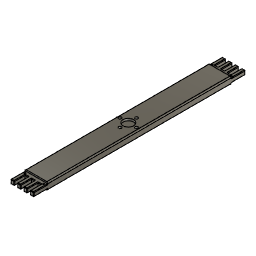
torsionbar_vFINAL v5 (Autodesk Fusion 360 design; units mm, degrees)
Autodesk Fusion 360 part; units mm, degrees
(part 1 of 5)
sketch "Sketch1" plane through (0, 0, 0) normal (0, 0, 1) x (1, 0, 0)
  line L0 (-15.999, -0.4) -> (-15.9943, 152)
  line L1 (16.0057, -0.4) -> (16.0057, 152)
  line L2 (16.0057, -0.4) -> (-15.999, -0.4)
  line L3 (-15.999, -0.4) -> (-15.9943, -152.8)
  line L4 (-15.9943, -152.8) -> (16.0057, -152.8)
  line L5 (16.0057, -0.4) -> (16.0057, -152.8)
  line L6 (16.0057, 152) -> (0.0057, 152)
  line L7 (0.0057, 152) -> (-15.9943, 152)
  dimension "d20" = 152.4
  dimension "d22" = 152.4
  dimension "d67" = 16
  dimension "d68" = 16
  constraint horizontal L2
  constraint symmetric L0.start L2 L3.start
  constraint symmetric L0.end L2 L3.end
  constraint symmetric L1.start L2 L5.start
  constraint symmetric L1.end L2 L4.end
  constraint vertical L1
  constraint perpendicular L1 L6
  constraint parallel L6 L7
  measures "d20" vertical distance of L0.start L0.end
  measures "d22" vertical distance of L1.start L1.end
  measures "d67" distance of L1.end L6.end
  measures "d68" distance of L0.end L6.end
extrude "Extrude3" add sketch "Sketch1" along normal blind 10
sketch "Sketch4" plane through (0, 0, 10) normal (0, 0, 1) x (-1, 0, 0)
  line L0 (15.999, 0.4) -> (15.9943, 152.8)
  line L1 (15.9943, 152.8) -> (-16.0057, 152.8)
  line L2 (-16.0057, 152.8) -> (-16.0057, -152)
  line L3 (15.9943, -152) -> (15.999, 0.4)
  circle A0 centre (0, 0) radius 7.5
  circle A1 centre (0, 11.5) radius 2
  circle A2 centre (-11.5, 0) radius 2
  circle A3 centre (0, -11.5) radius 2
  circle A4 centre (11.5, 0) radius 2
  line L4 (-16.0057, -152) -> (15.9943, -152)
  dimension "d36" = 15
  dimension "d50" = 4
  dimension "d51" = 4
  dimension "d52" = 4
  dimension "d53" = 4
  dimension "d54" = 11.5
  dimension "d55" = 11.5
  dimension "d56" = 11.5
  dimension "d57" = 11.5
  constraint coincident A0.centre origin
  measures "d36" diameter of A0
  measures "d50" diameter of A1
  measures "d51" diameter of A2
  measures "d52" diameter of A3
  measures "d53" diameter of A4
  measures "d54" distance of A0.centre A1.centre
  measures "d55" distance of A0.centre A4.centre
  measures "d56" distance of A0.centre A3.centre
  measures "d57" distance of A0.centre A2.centre
extrude "Extrude7" cut sketch "Sketch4" against normal blind 3 contours A0
extrude "Extrude9" cut sketch "Sketch4" against normal up to surface (10 mm away) contours A1 | A2 | A3 | A4
sketch "Sketch6" plane through (0, 152, 0) normal (0, 1, 0) x (-1, 0, 0)
  line L0 (-16.0057, 0) -> (15.9943, 0)
  line L1 (15.9943, 0) -> (15.9943, 10)
  line L2 (15.9943, 10) -> (-16.0057, 10)
  line L3 (-16.0057, 10) -> (-16.0057, 0)
  line L4 (10.9943, 8) -> (6.9943, 8)
  line L5 (1.9943, 8) -> (-2.0057, 8)
  line L6 (-7.0057, 8) -> (-11.0057, 8)
  line L7 (10.9943, 8) -> (10.9943, 2)
  line L8 (10.9943, 2) -> (6.9943, 2)
  line L9 (6.9943, 2) -> (6.9943, 8)
  line L10 (1.9943, 8) -> (1.9943, 2)
  line L11 (1.9943, 2) -> (-2.0057, 2)
  line L12 (-2.0057, 2) -> (-2.0057, 8)
  line L13 (-7.0057, 8) -> (-7.0057, 2)
  line L14 (-7.0057, 2) -> (-11.0057, 2)
  line L15 (-11.0057, 2) -> (-11.0057, 8)
  dimension "d78" = 4
  dimension "d79" = 4
  dimension "d80" = 4
  dimension "d95" = 6
  dimension "d96" = 4
  dimension "d97" = 4
  dimension "d98" = 4
  dimension "d99" = 5
  dimension "d100" = 5
  dimension "d101" = 2
  dimension "d102" = 2
  constraint perpendicular L4 L7
  constraint perpendicular L7 L8
  constraint perpendicular L5 L10
  constraint perpendicular L10 L11
  constraint perpendicular L6 L13
  constraint perpendicular L13 L14
  measures "d78" distance of L6.start L6.end
  measures "d79" distance of L5.start L5.end
  measures "d80" distance of L4.start L4.end
  measures "d95" distance of L4.start L7.end
  measures "d96" distance of L7.end L8.end
  measures "d97" distance of L10.end L11.end
  measures "d98" distance of L13.end L14.end
  measures "d99" distance of L12 L13
  measures "d100" distance of L9 L10
  measures "d101" distance of L0 L8
  measures "d102" distance of L0 L14
extrude "Extrude11" cut sketch "Sketch6" against normal blind 15 contours L4 L7 L8 L9 | L5 L10 L11 L12 | L6 L13 L14 L15
sketch "Sketch7" plane through (0, 0, 0) normal (0, 0, -1) x (1, 0, 0)
  line L0 (-15.9943, -152) -> (16.0057, -152)
  line L1 (16.0057, -152) -> (16.0057, 152.8)
  line L2 (16.0057, 152.8) -> (-15.9943, 152.8)
  line L3 (-15.9943, 152.8) -> (-15.999, 0.4)
  line L4 (-15.999, 0.4) -> (-15.9943, -152)
  circle A0 centre (11.5, 0) radius 2
  circle A1 centre (0, -11.5) radius 2
  circle A2 centre (0, 11.5) radius 2
  circle A3 centre (-11.5, 0) radius 2
  line L5 (-15.9949, -132) -> (16.0057, -132)
  line L6 (16.0057, -152) -> (-15.9943, -152)
  line L7 (-15.9949, -132) -> (-15.9943, -152)
  line L8 (16.0057, -152) -> (16.0057, -132)
  dimension "d94" = 20
  constraint coincident L4 L5.start
  constraint coincident L1 L5.end
  constraint perpendicular L1 L5
  constraint coincident L0.end L1.start
  constraint coincident L0.start L4.end
  constraint parallel L4 L7
  measures "d94" distance of L5 L6
extrude "Extrude12" cut sketch "Sketch7" against normal blind 2 contours L0 L1 L4 L5 L6 L7 L8
sketch "Sketch8" plane through (0, 0, 10) normal (0, 0, 1) x (-1, 0, 0)
  circle A0 centre (11.5, 0) radius 2
  circle A1 centre (0, 11.5) radius 2
  circle A2 centre (0, -11.5) radius 2
  circle A3 centre (-11.5, 0) radius 2
  circle A4 centre (0, 0) radius 7.5
  line L0 (-16.0057, -152) -> (15.9943, -152)
  line L1 (15.9943, -152) -> (15.999, 0.4)
  line L2 (15.999, 0.4) -> (15.9943, 152.8)
  line L3 (15.9943, 152.8) -> (-16.0057, 152.8)
  line L4 (-16.0057, 152.8) -> (-16.0057, -152)
  line L5 (15.9949, -132) -> (-16.0057, -132)
  line L6 (-16.0057, -152) -> (15.9943, -152)
  line L7 (-16.0057, -152) -> (-16.0057, -132)
  line L8 (15.9943, -152) -> (15.9949, -132)
  dimension "d91" = 20
  constraint coincident L1 L5.start
  constraint coincident L4 L5.end
  constraint perpendicular L4 L5
  constraint coincident L0.start L4.end
  constraint coincident L0.end L1.start
  measures "d91" distance of L5.end L0.start
extrude "Extrude13" cut sketch "Sketch8" against normal blind 2 contours L0 L1 L4 L5 L6 L7 L8
sketch "Sketch9" plane through (0, 0, 0) normal (0, 0, -1) x (1, 0, 0)
  line L0 (-15.9949, -132) -> (16.0057, -132)
  line L1 (16.0057, -132) -> (16.0057, 152.8)
  line L2 (16.0057, 152.8) -> (-15.9943, 152.8)
  line L3 (-15.9943, 152.8) -> (-15.999, 0.4)
  line L4 (-15.999, 0.4) -> (-15.9949, -132)
  circle A0 centre (-11.5, 0) radius 2
  circle A1 centre (0, 11.5) radius 2
  circle A2 centre (0, -11.5) radius 2
  circle A3 centre (11.5, 0) radius 2
sketch "Sketch10" plane through (0, 0, 0) normal (0, 0, -1) x (1, 0, 0)
  line L0 (-15.9949, -132) -> (16.0057, -132)
  line L1 (16.0057, -132) -> (16.0057, 152.8)
  line L2 (-15.9943, 152.8) -> (-15.999, 0.4)
  line L3 (-15.999, 0.4) -> (-15.9949, -132)
  circle A0 centre (-11.5, 0) radius 2
  circle A1 centre (0, 11.5) radius 2
  circle A2 centre (0, -11.5) radius 2
  circle A3 centre (11.5, 0) radius 2
  line L4 (16.0057, 132.8) -> (16.0057, 152.8)
  line L5 (16.0057, 152.8) -> (-17.8256, 152.8)
  line L6 (-17.8256, 152.8) -> (-17.8256, 132.8)
  line L7 (16.0057, 132.8) -> (-17.8256, 132.8)
  dimension "d112" = 20
  dimension "d119" = 20
  constraint coincident L1 L4.start
  constraint coincident L1.end L4.end
  constraint perpendicular L5 L6
  constraint perpendicular L6 L7
  measures "d112" distance of L4.start L1.end
  measures "d119" distance of L5.end L6.end
sketch "Sketch11" plane through (0, 0, 10) normal (0, 0, 1) x (-1, 0, 0)
  line L0 (-16.0057, -132) -> (15.9949, -132)
  line L1 (15.9949, -132) -> (15.999, 0.4)
  line L2 (15.999, 0.4) -> (15.9943, 152.8)
  line L3 (15.9943, 152.8) -> (-16.0057, 152.8)
  line L4 (-16.0057, 152.8) -> (-16.0057, -132)
  circle A0 centre (11.5, 0) radius 2
  circle A1 centre (0, 11.5) radius 2
  circle A2 centre (0, -11.5) radius 2
  circle A3 centre (-11.5, 0) radius 2
  circle A4 centre (0, 0) radius 7.5
  line L5 (-16.0057, 152.8) -> (-16.0057, 132.8)
  line L6 (-16.0057, 152.8) -> (15.9943, 152.8)
  line L7 (-16.0057, 132.8) -> (15.9949, 132.801)
  line L8 (15.9943, 152.8) -> (15.9949, 132.801)
  dimension "d114" = 20
  constraint coincident L3.end L4.start
  constraint coincident L4 L5.end
  constraint perpendicular L3 L5
  constraint coincident L2.end L3.start
  constraint coincident L2 L7.end
  constraint perpendicular L2 L7
  measures "d114" distance of L3.end L5.end
extrude "Extrude15" cut sketch "Sketch11" against normal blind 2 contours L2 L3 L4 L5 L6 L7 L8
extrude "Extrude16" cut sketch "Sketch10" against normal blind 2 contours L1 L2 L4 L5 L7
sketch "Sketch12" plane through (0, -152.8, 0) normal (0, -1, 0) x (1, 0, 0)
  line L0 (-15.9943, 2) -> (16.0057, 2)
  line L1 (16.0057, 2) -> (16.0057, 8)
  line L2 (16.0057, 8) -> (-15.9943, 8)
  line L3 (-15.9943, 8) -> (-15.9943, 2)
  line L4 (16.0057, 2) -> (11.0057, 2)
  line L5 (11.0057, 2) -> (7.0057, 2)
  line L6 (7.0057, 2) -> (2.0057, 2)
  line L7 (2.0057, 2) -> (-1.9943, 2)
  line L8 (-1.9943, 2) -> (-6.9943, 2)
  line L9 (-6.9943, 2) -> (-10.9943, 2)
  line L10 (-10.9943, 2) -> (-15.9943, 2)
  line L11 (11.0057, 2) -> (11.0057, 8)
  line L12 (7.0057, 2) -> (7.0057, 8)
  line L13 (2.0057, 2) -> (2.0057, 8)
  line L14 (-1.9943, 2) -> (-1.9943, 8)
  line L15 (-6.9943, 2) -> (-6.9943, 8)
  line L16 (-10.9943, 2) -> (-10.9943, 8)
  dimension "d120" = 5
  constraint coincident L0.end L1.start
  constraint perpendicular L1 L4
  constraint coincident L0 L5.end
  constraint parallel L0 L5
  constraint coincident L0 L6.end
  constraint parallel L0 L6
  constraint coincident L0 L7.end
  constraint coincident L0 L8.end
  constraint coincident L0 L9.end
  constraint parallel L0 L9
  constraint coincident L0.start L3.end
  constraint perpendicular L3 L10
  constraint coincident L2 L11.end
  constraint perpendicular L2 L11
  constraint coincident L2 L12.end
  constraint perpendicular L2 L12
  constraint perpendicular L6 L13
  constraint coincident L2 L14.end
  constraint perpendicular L2 L14
  constraint coincident L2 L15.end
  constraint perpendicular L2 L15
  constraint coincident L2 L16.end
  constraint perpendicular L2 L16
  measures "d120" distance of L0.end L4.end
extrude "Extrude17" cut sketch "Sketch12" against normal blind 15 contours L0 L2 L9 L15 L16 | L0 L2 L7 L13 L14 | L0 L2 L5 L11 L12
sketch "Sketch14" plane through (0, 0, 2) normal (0, 0, -1) x (1, 0, 0)
  line L0 (11.0057, 152.8) -> (11.0057, 137.8)
  line L1 (11.0057, 137.8) -> (7.0057, 137.8)
  line L2 (7.0057, 137.8) -> (7.0057, 152.8)
  line L3 (7.0057, 152.8) -> (2.0057, 152.8)
  line L4 (2.0057, 152.8) -> (2.0057, 137.8)
  line L5 (2.0057, 137.8) -> (-1.9943, 137.8)
  line L6 (-1.9943, 137.8) -> (-1.9943, 152.8)
  line L7 (-1.9943, 152.8) -> (-6.9943, 152.8)
  line L8 (-6.9943, 152.8) -> (-6.9943, 137.8)
  line L9 (-6.9943, 137.8) -> (-10.9943, 137.8)
  line L10 (-10.9943, 137.8) -> (-10.9943, 152.8)
  line L11 (-10.9943, 152.8) -> (-15.9943, 152.8)
  line L12 (-15.9943, 152.8) -> (-15.9949, 132.8)
  line L13 (-15.9949, 132.8) -> (16.0057, 132.8)
  line L14 (16.0057, 132.8) -> (16.0057, 152.8)
  line L15 (16.0057, 152.8) -> (11.0057, 152.8)
  circle A0 centre (13.0057, 135.8) radius 1
  circle A1 centre (-12.9948, 135.8) radius 1
  dimension "d132" = 3
  dimension "d133" = 3
  dimension "d134" = 3
  dimension "d135" = 3
  dimension "d136" = 2
  dimension "d137" = 2
  measures "d132" distance of L13 A1.centre
  measures "d133" distance of L12 A1.centre
  measures "d134" distance of L14 A0.centre
  measures "d135" distance of L13 A0.centre
  measures "d136" diameter of A0
  measures "d137" diameter of A1
extrude "Extrude19" cut sketch "Sketch14" against normal up to surface (6 mm away) contours A0 | A1
sketch "Sketch15" plane through (0, 0, 2) normal (0, 0, -1) x (1, 0, 0)
  line L0 (7.0057, -152) -> (7.0057, -137)
  line L1 (7.0057, -137) -> (11.0057, -137)
  line L2 (11.0057, -137) -> (11.0057, -152)
  line L3 (11.0057, -152) -> (16.0057, -152)
  line L4 (16.0057, -152) -> (16.0057, -132)
  line L5 (16.0057, -132) -> (-15.9949, -132)
  line L6 (-15.9949, -132) -> (-15.9943, -152)
  line L7 (-15.9943, -152) -> (-10.9943, -152)
  line L8 (-10.9943, -152) -> (-10.9943, -137)
  line L9 (-10.9943, -137) -> (-6.9943, -137)
  line L10 (-6.9943, -137) -> (-6.9943, -152)
  line L11 (-6.9943, -152) -> (-1.9943, -152)
  line L12 (-1.9943, -152) -> (-1.9943, -137)
  line L13 (-1.9943, -137) -> (2.0057, -137)
  line L14 (2.0057, -137) -> (2.0057, -152)
  line L15 (2.0057, -152) -> (7.0057, -152)
  circle A0 centre (-12.9948, -135) radius 1
  circle A1 centre (13.0057, -135) radius 1
  dimension "d140" = 2
  dimension "d141" = 2
  dimension "d142" = 3
  dimension "d143" = 3
  dimension "d144" = 3
  dimension "d145" = 3
  measures "d140" diameter of A0
  measures "d141" diameter of A1
  measures "d142" distance of L6 A0.centre
  measures "d143" distance of L4 A1.centre
  measures "d144" distance of L5 A0.centre
  measures "d145" distance of L5 A1.centre
extrude "Extrude20" cut sketch "Sketch15" against normal up to surface (6 mm away) contours A0 | A1
move_face "OffsetFaces1" offset -5 2 faces at (5.3389, -132.8003, 9.3333) (5.3389, -132.8, 1.3333)
move_face "OffsetFaces2" offset -5 4 faces at (12.6724, -152.8, 4) (3.6724, -152.8, 4) (-5.3276, -152.8, 4) (-14.3276, -152.8, 4)
extrude "Extrude21" cut 3 faces at (-9.6609, -137.8, 6) (0.6724, -137.8, 4) (8.3391, -137.8, 6) along direction (0, 1, 0) blind 5
move_face "MoveFace1" to x (1, 0, 0) y (0, 1, 0) z (0, 0, 1) at (0, 5, 0) 2 faces at (13.9748, -136.0468, 6) (-12.0257, -136.0468, 6)
fillet "Fillet1" radius 0.7937 4 faces at (-14.3277, -147.8, 4) (-5.3276, -147.8, 4) (3.6724, -147.8, 4) (12.6724, -147.8, 4)
fillet "Fillet2" radius 0.7937 17 edges at (-15.762, -147.5675, 7.7675) (-15.9944, -147.0063, 8) (-15.9947, -137.4036, 8) (-11.2268, -147.5675, 7.7675) (-10.9943, -139.9031, 8) (-6.9943, -139.9031, 8) (-6.7618, -147.5675, 7.7675) (-2.2268, -147.5675, 7.7675) (-1.9943, -139.9031, 8) (2.0057, -139.9031, 8) (2.2382, -147.5675, 7.7675) (6.7732, -147.5675, 7.7675) (7.0057, -139.9031, 8) (11.0057, -139.9031, 8) (11.2382, -147.5675, 7.7675) (16.0057, -137.4031, 8) (15.7732, -147.5675, 7.7675)
fillet "Fillet3" radius 0.7937 3 edges at (-8.9943, -132.8, 8) (0.0057, -132.8, 8) (9.0057, -132.8, 8)
fillet "Fillet4" radius 0.7937 20 edges at (-15.9947, -137.4031, 2) (-15.9944, -147.0063, 2) (-15.762, -147.5675, 2.2325) (-10.9943, -139.9031, 2) (-11.2268, -147.5675, 2.2325) (-8.9943, -132.8, 2) (-6.7618, -147.5675, 2.2325) (-6.9943, -139.9031, 2) (-1.9943, -139.9031, 2) (-2.2268, -147.5675, 2.2325) (0.0057, -132.8, 2) (2.2382, -147.5675, 2.2325) (2.0057, -139.9031, 2) (7.0057, -139.9031, 2) (6.7732, -147.5675, 2.2325) (9.0057, -132.8, 2) (11.2382, -147.5675, 2.2325) (11.0057, -139.9031, 2) (15.7732, -147.5675, 2.2325) (16.0057, -137.4031, 2)
extrude "Extrude22" cut 2 faces at (-5.328, 132, 8.6667) (-5.328, 132, 0.6667) along direction (0, -1, 0) blind 5
extrude "Extrude23" cut 4 faces at (12.6724, 152, 4) (3.6724, 152, 4) (-5.3276, 152, 4) (-14.3276, 152, 6) along direction (0, -1, 0) blind 5
extrude "Extrude24" cut 3 faces at (9.6724, 137, 6) (0.6724, 137, 6) (-8.3276, 137, 6) along direction (0, -1, 0) blind 5
move_face "MoveFace2" to x (1, 0, 0) y (0, 1, 0) z (0, 0, 1) at (0, -5, 0) 2 faces at (-12.0257, 134.7532, 6) (13.9748, 134.7532, 6)
extrude "Extrude25" cut 1 faces at (-15.9949, 130.3333, 8.6667) along direction (-1, 0, 0) blind 3
extrude "Extrude26" cut 1 faces at (-15.9943, 150.3333, 4) along direction (-1, 0, 0) blind 5
extrude "Extrude27" cut 1 faces at (-15.9949, 130.3333, 1.3333) along direction (-1, 0, 0) blind 5
fillet "Fillet5" radius 0.7937 11 edges at (16.0057, 137, 8) (11.0057, 139.5, 8) (9.0057, 132, 8) (7.0057, 139.5, 8) (2.0057, 139.5, 8) (0.0057, 132, 8) (-1.9943, 139.5, 8) (-6.9943, 139.5, 8) (-8.9943, 132, 8) (-10.9943, 139.5, 8) (-15.9947, 137, 8) 4 faces at (12.6724, 147, 4) (3.6724, 147, 4) (-5.3276, 147, 4) (-12.661, 147, 4)
fillet "Fillet6" radius 0.7937 20 edges at (16.0057, 136.6031, 2) (15.7732, 146.7675, 2.2325) (11.2382, 146.7675, 2.2325) (11.0057, 139.1031, 2) (9.0057, 132, 2) (6.7732, 146.7675, 2.2325) (7.0057, 139.1031, 2) (2.2382, 146.7675, 2.2325) (2.0057, 139.1031, 2) (0.0057, 132, 2) (-2.2268, 146.7675, 2.2325) (-1.9943, 139.1031, 2) (-6.7618, 146.7675, 2.2325) (-6.9943, 139.1031, 2) (-8.9943, 132, 2) (-11.2268, 146.7675, 2.2325) (-10.9943, 139.1031, 2) (-15.762, 146.7675, 2.2325) (-15.9944, 146.2063, 2) (-15.9947, 136.6031, 2)
fillet "Fillet7" radius 1.5875 6 edges at (16.0057, -0.4, 10) (-15.997, 63.3, 10) (-15.997, -64.1005, 10) (16.0057, -0.4, 0) (-15.997, -64.1, 0) (-15.997, 63.3, 0)
sketch "Sketch16" plane through (0, 0, 0) normal (0, 0, -1) x (1, 0, 0)
  line L0 (-14.4115, 0.4) -> (-14.4075, -127)
  line L1 (-14.4075, -127) -> (14.4182, -127)
  line L2 (14.4182, -127) -> (14.4182, 127.8)
  line L3 (14.4182, 127.8) -> (-14.4075, 127.8)
  line L4 (-14.4075, 127.8) -> (-14.4115, 0.4)
  circle A0 centre (-11.5, 0) radius 2
  circle A1 centre (0, 11.5) radius 2
  circle A2 centre (0, -11.5) radius 2
  circle A3 centre (11.5, 0) radius 2
  spline S0 degree 3 poles (-41.1368, -32.0875) (-41.0058, -32.6966) (-40.9336, -32.8566) (-40.2646, -34.0174) knots 0 0 0 0 1 1 1 1
  spline S1 degree 3 poles (-40.2646, -34.0174) (-40.0221, -34.4378) (-39.6654, -35.0569) (-39.4721, -35.3933) knots 0 0 0 0 1 1 1 1
  spline S2 degree 3 poles (-39.4721, -35.3933) (-39.1408, -35.9687) (-37.9129, -38.0978) (-36.7496, -40.1131) knots 0 0 0 0 1 1 1 1
  spline S3 degree 3 poles (-36.7496, -40.1131) (-36.4645, -40.607) (-36.1508, -41.1487) (-36.0521, -41.3169) knots 0 0 0 0 1 1 1 1
  spline S4 degree 3 poles (-36.0521, -41.3169) (-35.9534, -41.4851) (-35.5661, -42.1558) (-35.1915, -42.8073) knots 0 0 0 0 1 1 1 1
  spline S5 degree 3 poles (-35.1915, -42.8073) (-33.8969, -45.0592) (-33.2409, -45.6532) (-31.7334, -45.939) knots 0 0 0 0 1 1 1 1
  spline S6 degree 3 poles (-31.7334, -45.939) (-31.2535, -46.0302) (-18.2743, -46.0292) (-17.8306, -45.938) knots 0 0 0 0 1 1 1 1
  spline S7 degree 3 poles (-17.8306, -45.938) (-16.7915, -45.7247) (-15.8703, -45.1366) (-15.265, -44.2997) knots 0 0 0 0 1 1 1 1
  spline S8 degree 3 poles (-15.265, -44.2997) (-15.1343, -44.1188) (-14.6091, -43.2366) (-14.6242, -43.2231) knots 0 0 0 0 1 1 1 1
  spline S9 degree 3 poles (-14.6242, -43.2231) (-14.6314, -43.2166) (-15.4033, -43.0993) (-15.5443, -43.0832) knots 0 0 0 0 1 1 1 1
  spline S10 degree 3 poles (-15.5443, -43.0832) (-15.5972, -43.077) (-15.6633, -43.1537) (-15.7926, -43.37) knots 0 0 0 0 1 1 1 1
  spline S11 degree 3 poles (-15.7926, -43.37) (-16.2858, -44.1959) (-16.8785, -44.6712) (-17.7659, -44.9533) knots 0 0 0 0 1 1 1 1
  line L5 (-17.7659, -44.9533) -> (-18.1092, -45.0623)
  line L6 (-18.1092, -45.0623) -> (-24.7782, -45.0623)
  line L7 (-24.7782, -45.0623) -> (-31.4472, -45.0623)
  line L8 (-31.4472, -45.0623) -> (-31.7451, -44.976)
  spline S12 degree 3 poles (-31.7451, -44.976) (-32.8681, -44.6502) (-33.2526, -44.2667) (-34.332, -42.3952) knots 0 0 0 0 1 1 1 1
  spline S13 degree 3 poles (-34.332, -42.3952) (-34.7592, -41.655) (-35.1891, -40.9117) (-35.2875, -40.7435) knots 0 0 0 0 1 1 1 1
  spline S14 degree 3 poles (-35.2875, -40.7435) (-35.3862, -40.5754) (-35.6349, -40.1454) (-35.8406, -39.788) knots 0 0 0 0 1 1 1 1
  spline S15 degree 3 poles (-35.8406, -39.788) (-36.0459, -39.431) (-36.2791, -39.0269) (-36.3586, -38.89) knots 0 0 0 0 1 1 1 1
  spline S16 degree 3 poles (-36.3586, -38.89) (-36.4384, -38.7534) (-37.0482, -37.6957) (-37.7141, -36.5397) knots 0 0 0 0 1 1 1 1
  spline S17 degree 3 poles (-37.7141, -36.5397) (-38.38, -35.3836) (-39.0153, -34.283) (-39.1264, -34.0938) knots 0 0 0 0 1 1 1 1
  spline S18 degree 3 poles (-39.1264, -34.0938) (-40.193, -32.2729) (-40.3344, -31.8983) (-40.2835, -31.0315) knots 0 0 0 0 1 1 1 1
  spline S19 degree 3 poles (-40.2835, -31.0315) (-40.2453, -30.3825) (-40.127, -30.074) (-39.4979, -28.9846) knots 0 0 0 0 1 1 1 1
  line L9 (-39.4979, -28.9846) -> (-39.1295, -28.3469)
  line L10 (-39.1295, -28.3469) -> (-39.0865, -28.5451)
  spline S20 degree 3 poles (-39.0865, -28.5451) (-39.0628, -28.6541) (-38.9981, -28.9496) (-38.9431, -29.202) knots 0 0 0 0 1 1 1 1
  spline S21 degree 3 poles (-38.9431, -29.202) (-38.747, -30.0991) (-38.3429, -31.2854) (-37.9968, -31.9795) knots 0 0 0 0 1 1 1 1
  line L11 (-37.9968, -31.9795) -> (-37.8507, -32.2729)
  line L12 (-37.8507, -32.2729) -> (-38.1165, -32.1993)
  spline S22 degree 3 poles (-38.1165, -32.1993) (-38.2631, -32.1587) (-38.3938, -32.1257) (-38.4075, -32.1257) knots 0 0 0 0 1 1 1 1
  spline S23 degree 3 poles (-38.4075, -32.1257) (-38.4213, -32.1257) (-38.423, -32.276) (-38.4113, -32.46) knots 0 0 0 0 1 1 1 1
  spline S24 degree 3 poles (-38.4113, -32.46) (-38.3178, -33.9425) (-36.1488, -36.8162) (-33.8222, -38.5415) knots 0 0 0 0 1 1 1 1
  line L13 (-33.8222, -38.5415) -> (-33.4838, -38.7926)
  line L14 (-33.4838, -38.7926) -> (-33.7073, -38.9818)
  spline S25 degree 3 poles (-33.7073, -38.9818) (-34.925, -40.0116) (-34.938, -40.3026) (-33.7785, -40.5709) knots 0 0 0 0 1 1 1 1
  spline S26 degree 3 poles (-33.7785, -40.5709) (-32.6995, -40.8203) (-32.0536, -40.8065) (-31.4998, -40.5224) knots 0 0 0 0 1 1 1 1
  line L15 (-31.4998, -40.5224) -> (-31.247, -40.3927)
  line L16 (-31.247, -40.3927) -> (-31.0303, -40.5203)
  spline S27 degree 3 poles (-31.0303, -40.5203) (-30.7459, -40.6878) (-30.5013, -40.8705) (-30.0139, -41.2801) knots 0 0 0 0 1 1 1 1
  spline S28 degree 3 poles (-30.0139, -41.2801) (-28.6677, -42.4117) (-26.9489, -42.9363) (-25.5043, -42.6566) knots 0 0 0 0 1 1 1 1
  spline S29 degree 3 poles (-25.5043, -42.6566) (-24.8755, -42.5349) (-20.997, -42.4671) (-19.7719, -42.5569) knots 0 0 0 0 1 1 1 1
  spline S30 degree 3 poles (-19.7719, -42.5569) (-19.4881, -42.5775) (-18.5178, -42.5951) (-17.6159, -42.5958) knots 0 0 0 0 1 1 1 1
  spline S31 degree 3 poles (-17.6159, -42.5958) (-16.0647, -42.5971) (-15.9343, -42.6026) (-15.2082, -42.6986) knots 0 0 0 0 1 1 1 1
  spline S32 degree 3 poles (-15.2082, -42.6986) (-14.1585, -42.8369) (-13.4705, -42.8358) (-12.6822, -42.6948) knots 0 0 0 0 1 1 1 1
  spline S33 degree 3 poles (-12.6822, -42.6948) (-11.4467, -42.4737) (-11.447, -42.4737) (-10.9435, -42.5032) knots 0 0 0 0 1 1 1 1
  spline S34 degree 3 poles (-10.9435, -42.5032) (-10.0489, -42.5555) (-9.9935, -42.5517) (-9.7586, -42.4176) knots 0 0 0 0 1 1 1 1
  spline S35 degree 3 poles (-9.7586, -42.4176) (-9.643, -42.3516) (-9.4376, -42.269) (-9.3018, -42.2343) knots 0 0 0 0 1 1 1 1
  spline S36 degree 3 poles (-9.3018, -42.2343) (-8.7215, -42.0846) (-8.543, -41.8549) (-8.3824, -41.0493) knots 0 0 0 0 1 1 1 1
  spline S37 degree 3 poles (-8.3824, -41.0493) (-8.283, -40.5527) (-8.2771, -40.5396) (-8.0167, -40.2572) knots 0 0 0 0 1 1 1 1
  spline S38 degree 3 poles (-8.0167, -40.2572) (-7.4798, -39.6745) (-7.3873, -38.9687) (-7.7708, -38.3874) knots 0 0 0 0 1 1 1 1
  line L17 (-7.7708, -38.3874) -> (-7.9136, -38.1711)
  line L18 (-7.9136, -38.1711) -> (-7.7564, -38.0139)
  line L19 (-7.7564, -38.0139) -> (-7.5995, -37.8567)
  line L20 (-7.5995, -37.8567) -> (-7.6033, -37.4464)
  spline S39 degree 3 poles (-7.6033, -37.4464) (-7.6085, -36.8706) (-7.6886, -36.6694) (-8.0611, -36.2993) knots 0 0 0 0 1 1 1 1
  spline S40 degree 3 poles (-8.0611, -36.2993) (-8.6661, -35.6977) (-10.0413, -35.3479) (-10.6611, -35.6378) knots 0 0 0 0 1 1 1 1
  spline S41 degree 3 poles (-10.6611, -35.6378) (-11.2603, -35.9185) (-11.7208, -35.7926) (-12.817, -35.049) knots 0 0 0 0 1 1 1 1
  spline S42 degree 3 poles (-12.817, -35.049) (-14.3645, -33.9992) (-15.4459, -33.4908) (-16.6188, -33.2614) knots 0 0 0 0 1 1 1 1
  line L21 (-16.6188, -33.2614) -> (-17.0773, -33.1716)
  line L22 (-17.0773, -33.1716) -> (-17.2304, -32.8948)
  spline S43 degree 3 poles (-17.2304, -32.8948) (-17.792, -31.878) (-19.2869, -30.9442) (-20.8185, -30.6535) knots 0 0 0 0 1 1 1 1
  spline S44 degree 3 poles (-20.8185, -30.6535) (-21.2585, -30.5703) (-21.4256, -30.4179) (-21.9729, -29.6031) knots 0 0 0 0 1 1 1 1
  spline S45 degree 3 poles (-21.9729, -29.6031) (-22.4293, -28.9231) (-22.4795, -28.2713) (-22.1369, -27.4723) knots 0 0 0 0 1 1 1 1
  spline S46 degree 3 poles (-22.1369, -27.4723) (-21.752, -26.5738) (-19.7908, -24.7622) (-18.1078, -23.7503) knots 0 0 0 0 1 1 1 1
  spline S47 degree 3 poles (-18.1078, -23.7503) (-17.4016, -23.3255) (-17.4023, -23.3258) (-15.9691, -23.3148) knots 0 0 0 0 1 1 1 1
  spline S48 degree 3 poles (-15.9691, -23.3148) (-14.8271, -23.3062) (-14.5145, -23.2859) (-13.6167, -23.1604) knots 0 0 0 0 1 1 1 1
  line L23 (-13.6167, -23.1604) -> (-13.4427, -23.136)
  line L24 (-13.4427, -23.136) -> (-13.0378, -23.8376)
  spline S49 degree 3 poles (-13.0378, -23.8376) (-12.8153, -24.2236) (-11.9919, -25.6486) (-11.208, -27.0045) knots 0 0 0 0 1 1 1 1
  spline S50 degree 3 poles (-11.208, -27.0045) (-9.2643, -30.3663) (-9.2952, -30.2989) (-9.2897, -31.1891) knots 0 0 0 0 1 1 1 1
  spline S51 degree 3 poles (-9.2897, -31.1891) (-9.2849, -31.9699) (-9.3812, -32.2478) (-10.0719, -33.4503) knots 0 0 0 0 1 1 1 1
  spline S52 degree 3 poles (-10.0719, -33.4503) (-11.1712, -35.3634) (-11.1041, -35.2351) (-11.0322, -35.288) knots 0 0 0 0 1 1 1 1
  spline S53 degree 3 poles (-11.0322, -35.288) (-10.9318, -35.3616) (-10.8186, -35.3458) (-10.5552, -35.2213) knots 0 0 0 0 1 1 1 1
  spline S54 degree 3 poles (-10.5552, -35.2213) (-10.387, -35.1418) (-10.2542, -35.1064) (-10.1218, -35.1064) knots 0 0 0 0 1 1 1 1
  spline S55 degree 3 poles (-10.1218, -35.1064) (-9.9467, -35.1061) (-9.9247, -35.0958) (-9.859, -34.9822) knots 0 0 0 0 1 1 1 1
  spline S56 degree 3 poles (-9.859, -34.9822) (-9.8194, -34.9138) (-9.6285, -34.5829) (-9.4345, -34.2465) knots 0 0 0 0 1 1 1 1
  spline S57 degree 3 poles (-9.4345, -34.2465) (-9.2406, -33.9105) (-9.0256, -33.5407) (-8.9564, -33.4248) knots 0 0 0 0 1 1 1 1
  spline S58 degree 3 poles (-8.9564, -33.4248) (-8.371, -32.4449) (-8.1915, -31.2372) (-8.4718, -30.1672) knots 0 0 0 0 1 1 1 1
  spline S59 degree 3 poles (-8.4718, -30.1672) (-8.6152, -29.6199) (-8.6837, -29.4858) (-9.8291, -27.5012) knots 0 0 0 0 1 1 1 1
  spline S60 degree 3 poles (-9.8291, -27.5012) (-10.4055, -26.5026) (-10.9806, -25.5052) (-11.1072, -25.2847) knots 0 0 0 0 1 1 1 1
  spline S61 degree 3 poles (-11.1072, -25.2847) (-11.4594, -24.6711) (-11.7074, -24.2415) (-12.0115, -23.7176) knots 0 0 0 0 1 1 1 1
  spline S62 degree 3 poles (-12.0115, -23.7176) (-12.1642, -23.4548) (-12.5904, -22.7153) (-12.9587, -22.0742) knots 0 0 0 0 1 1 1 1
  spline S63 degree 3 poles (-12.9587, -22.0742) (-13.3271, -21.4334) (-13.7096, -20.7713) (-13.809, -20.6031) knots 0 0 0 0 1 1 1 1
  spline S64 degree 3 poles (-13.809, -20.6031) (-13.9084, -20.4349) (-14.2369, -19.8673) (-14.5392, -19.3418) knots 0 0 0 0 1 1 1 1
  spline S65 degree 3 poles (-14.5392, -19.3418) (-15.6815, -17.3554) (-16.41, -16.7394) (-17.931, -16.4742) knots 0 0 0 0 1 1 1 1
  spline S66 degree 3 poles (-17.931, -16.4742) (-18.4139, -16.3899) (-31.0671, -16.3899) (-31.5473, -16.4742) knots 0 0 0 0 1 1 1 1
  spline S67 degree 3 poles (-31.5473, -16.4742) (-32.627, -16.6637) (-33.6389, -17.2746) (-34.2707, -18.1187) knots 0 0 0 0 1 1 1 1
  spline S68 degree 3 poles (-34.2707, -18.1187) (-34.5019, -18.4272) (-34.6157, -18.6164) (-35.5269, -20.2017) knots 0 0 0 0 1 1 1 1
  spline S69 degree 3 poles (-35.5269, -20.2017) (-36.1553, -21.2944) (-36.4769, -21.8523) (-37.5989, -23.794) knots 0 0 0 0 1 1 1 1
  spline S70 degree 3 poles (-37.5989, -23.794) (-37.8479, -24.2249) (-38.2008, -24.8355) (-38.3828, -25.1509) knots 0 0 0 0 1 1 1 1
  spline S71 degree 3 poles (-38.3828, -25.1509) (-38.5647, -25.4663) (-38.8829, -26.0166) (-39.0896, -26.3737) knots 0 0 0 0 1 1 1 1
  spline S72 degree 3 poles (-39.0896, -26.3737) (-41.0027, -29.6784) (-41.0209, -29.7145) (-41.1523, -30.4055) knots 0 0 0 0 1 1 1 1
  spline S73 degree 3 poles (-41.1523, -30.4055) (-41.2349, -30.8413) (-41.2273, -31.6655) (-41.1368, -32.0875) knots 0 0 0 0 1 1 1 1
  line L25 (-38.5692, -27.3639) -> (-38.4491, -27.1658)
  line L26 (-38.4491, -27.1658) -> (-38.1967, -27.3288)
  spline S74 degree 3 poles (-38.1967, -27.3288) (-37.593, -27.7182) (-36.4016, -28.209) (-35.7848, -28.3222) knots 0 0 0 0 1 1 1 1
  line L27 (-35.7848, -28.3222) -> (-35.651, -28.3469)
  line L28 (-35.651, -28.3469) -> (-35.6631, -28.7735)
  spline S75 degree 3 poles (-35.6631, -28.7735) (-35.6971, -29.9666) (-35.5964, -30.7227) (-35.2686, -31.7377) knots 0 0 0 0 1 1 1 1
  spline S76 degree 3 poles (-35.2686, -31.7377) (-35.1712, -32.039) (-35.0976, -32.2918) (-35.1052, -32.2994) knots 0 0 0 0 1 1 1 1
  spline S77 degree 3 poles (-35.1052, -32.2994) (-35.1809, -32.375) (-37.0764, -32.417) (-37.1703, -32.3455) knots 0 0 0 0 1 1 1 1
  spline S78 degree 3 poles (-37.1703, -32.3455) (-37.4702, -32.1157) (-38.1908, -30.1899) (-38.4749, -28.8581) knots 0 0 0 0 1 1 1 1
  spline S79 degree 3 poles (-38.4749, -28.8581) (-38.7188, -27.7151) (-38.725, -27.6209) (-38.5692, -27.3639) knots 0 0 0 0 1 1 1 1
  spline S80 degree 3 poles (-37.8527, -26.1277) (-37.7705, -25.9898) (-37.3818, -25.318) (-36.9884, -24.6349) knots 0 0 0 0 1 1 1 1
  spline S81 degree 3 poles (-36.9884, -24.6349) (-36.5952, -23.9518) (-36.0741, -23.0483) (-35.8306, -22.6269) knots 0 0 0 0 1 1 1 1
  line L29 (-35.8306, -22.6269) -> (-35.3876, -21.8613)
  line L30 (-35.3876, -21.8613) -> (-35.0952, -22.0535)
  line L31 (-35.0952, -22.0535) -> (-34.8028, -22.2462)
  line L32 (-34.8028, -22.2462) -> (-34.8923, -22.5327)
  spline S82 degree 3 poles (-34.8923, -22.5327) (-35.1038, -23.212) (-35.3484, -24.927) (-35.5609, -27.2243) knots 0 0 0 0 1 1 1 1
  spline S83 degree 3 poles (-35.5609, -27.2243) (-35.616, -27.8193) (-35.5403, -27.7794) (-36.2657, -27.5954) knots 0 0 0 0 1 1 1 1
  spline S84 degree 3 poles (-36.2657, -27.5954) (-37.3887, -27.3103) (-37.7368, -27.1926) (-37.7805, -27.0843) knots 0 0 0 0 1 1 1 1
  spline S85 degree 3 poles (-37.7805, -27.0843) (-37.8152, -26.9983) (-37.9917, -26.4418) (-37.9989, -26.3953) knots 0 0 0 0 1 1 1 1
  spline S86 degree 3 poles (-37.9989, -26.3953) (-38.0003, -26.386) (-37.9346, -26.2657) (-37.8527, -26.1277) knots 0 0 0 0 1 1 1 1
  spline S87 degree 3 poles (-37.82, -32.5253) (-37.3131, -32.7204) (-36.222, -32.8899) (-35.4722, -32.8899) knots 0 0 0 0 1 1 1 1
  line L33 (-35.4722, -32.8899) -> (-34.8868, -32.8903)
  line L34 (-34.8868, -32.8903) -> (-34.7585, -33.2628)
  spline S88 degree 3 poles (-34.7585, -33.2628) (-34.3313, -34.5021) (-33.7507, -35.7754) (-32.7191, -37.736) knots 0 0 0 0 1 1 1 1
  spline S89 degree 3 poles (-32.7191, -37.736) (-32.5719, -38.016) (-32.4577, -38.2498) (-32.4653, -38.2564) knots 0 0 0 0 1 1 1 1
  spline S90 degree 3 poles (-32.4653, -38.2564) (-32.4729, -38.2626) (-32.6067, -38.3059) (-32.7625, -38.3527) knots 0 0 0 0 1 1 1 1
  line L35 (-32.7625, -38.3527) -> (-33.0459, -38.4377)
  line L36 (-33.0459, -38.4377) -> (-33.2784, -38.2753)
  spline S91 degree 3 poles (-33.2784, -38.2753) (-34.1366, -37.6761) (-35.5035, -36.3939) (-36.177, -35.556) knots 0 0 0 0 1 1 1 1
  spline S92 degree 3 poles (-36.177, -35.556) (-37.1125, -34.392) (-38.2046, -32.3771) (-37.82, -32.5253) knots 0 0 0 0 1 1 1 1
  spline S93 degree 3 poles (-36.2846, -28.9946) (-36.0641, -29.2151) (-35.7291, -29.0775) (-35.7291, -28.7666) knots 0 0 0 0 1 1 1 1
  spline S94 degree 3 poles (-35.7291, -28.7666) (-35.7291, -28.5537) (-35.8437, -28.4391) (-36.0566, -28.4391) knots 0 0 0 0 1 1 1 1
  spline S95 degree 3 poles (-36.0566, -28.4391) (-36.3675, -28.4391) (-36.5051, -28.7741) (-36.2846, -28.9946) knots 0 0 0 0 1 1 1 1
  spline S96 degree 3 poles (-35.5781, -22.7817) (-35.4498, -22.9097) (-35.3202, -22.9341) (-35.163, -22.8594) knots 0 0 0 0 1 1 1 1
  spline S97 degree 3 poles (-35.163, -22.8594) (-34.7612, -22.6689) (-34.9676, -22.0886) (-35.4058, -22.1763) knots 0 0 0 0 1 1 1 1
  spline S98 degree 3 poles (-35.4058, -22.1763) (-35.6596, -22.2269) (-35.7642, -22.5953) (-35.5781, -22.7817) knots 0 0 0 0 1 1 1 1
  spline S99 degree 3 poles (-35.4357, -33.5909) (-35.4134, -33.6298) (-35.336, -33.6862) (-35.2637, -33.7161) knots 0 0 0 0 1 1 1 1
  spline S100 degree 3 poles (-35.2637, -33.7161) (-34.9033, -33.8668) (-34.6298, -33.3663) (-34.9501, -33.1421) knots 0 0 0 0 1 1 1 1
  spline S101 degree 3 poles (-34.9501, -33.1421) (-35.2428, -32.9371) (-35.6156, -33.2817) (-35.4357, -33.5909) knots 0 0 0 0 1 1 1 1
  spline S102 degree 3 poles (-34.9848, -26.7751) (-34.6825, -23.9071) (-34.5913, -23.3551) (-34.2422, -22.283) knots 0 0 0 0 1 1 1 1
  spline S103 degree 3 poles (-34.2422, -22.283) (-34.1053, -21.8633) (-33.9244, -21.2879) (-33.8394, -21.0041) knots 0 0 0 0 1 1 1 1
  spline S104 degree 3 poles (-33.8394, -21.0041) (-33.6248, -20.2852) (-32.9733, -18.325) (-32.8911, -18.1493) knots 0 0 0 0 1 1 1 1
  spline S105 degree 3 poles (-32.8911, -18.1493) (-32.7498, -17.8486) (-31.8799, -17.4555) (-31.1761, -17.375) knots 0 0 0 0 1 1 1 1
  spline S106 degree 3 poles (-31.1761, -17.375) (-30.9705, -17.3513) (-29.5334, -17.3358) (-27.546, -17.3358) knots 0 0 0 0 1 1 1 1
  line L37 (-27.546, -17.3358) -> (-24.2564, -17.3355)
  line L38 (-24.2564, -17.3355) -> (-24.8934, -17.9945)
  spline S107 degree 3 poles (-24.8934, -17.9945) (-25.7134, -18.8437) (-25.9239, -19.0821) (-26.1268, -19.393) knots 0 0 0 0 1 1 1 1
  spline S108 degree 3 poles (-26.1268, -19.393) (-26.9523, -20.6595) (-27.9385, -23.5181) (-28.6525, -26.7176) knots 0 0 0 0 1 1 1 1
  spline S109 degree 3 poles (-28.6525, -26.7176) (-28.8018, -27.3876) (-28.9958, -28.532) (-28.9652, -28.563) knots 0 0 0 0 1 1 1 1
  spline S110 degree 3 poles (-28.9652, -28.563) (-28.9418, -28.5863) (-28.9415, -28.5853) (-28.7736, -28.0449) knots 0 0 0 0 1 1 1 1
  spline S111 degree 3 poles (-28.7736, -28.0449) (-28.1304, -25.975) (-26.3528, -22.2111) (-25.3798, -20.8579) knots 0 0 0 0 1 1 1 1
  spline S112 degree 3 poles (-25.3798, -20.8579) (-24.8876, -20.1735) (-23.9905, -19.4302) (-22.1221, -18.1586) knots 0 0 0 0 1 1 1 1
  spline S113 degree 3 poles (-22.1221, -18.1586) (-21.8487, -17.9725) (-21.4824, -17.7097) (-21.308, -17.5742) knots 0 0 0 0 1 1 1 1
  line L39 (-21.308, -17.5742) -> (-20.9909, -17.3282)
  line L40 (-20.9909, -17.3282) -> (-19.5882, -17.3454)
  spline S114 degree 3 poles (-19.5882, -17.3454) (-17.1609, -17.375) (-16.5999, -17.6698) (-15.5659, -19.4563) knots 0 0 0 0 1 1 1 1
  spline S115 degree 3 poles (-15.5659, -19.4563) (-14.4006, -21.4702) (-13.8929, -22.3597) (-13.9029, -22.3707) knots 0 0 0 0 1 1 1 1
  spline S116 degree 3 poles (-13.9029, -22.3707) (-13.9676, -22.4405) (-15.2653, -22.5729) (-16.2367, -22.609) knots 0 0 0 0 1 1 1 1
  spline S117 degree 3 poles (-16.2367, -22.609) (-17.692, -22.663) (-18.1222, -22.8498) (-19.6976, -24.1132) knots 0 0 0 0 1 1 1 1
  line L41 (-19.6976, -24.1132) -> (-20.1014, -24.4368)
  line L42 (-20.1014, -24.4368) -> (-20.4237, -24.399)
  spline S118 degree 3 poles (-20.4237, -24.399) (-21.7672, -24.2415) (-23.2586, -24.7622) (-24.1749, -25.7088) knots 0 0 0 0 1 1 1 1
  spline S119 degree 3 poles (-24.1749, -25.7088) (-24.9863, -26.5467) (-26.2792, -28.6152) (-26.7401, -29.8132) knots 0 0 0 0 1 1 1 1
  spline S120 degree 3 poles (-26.7401, -29.8132) (-27.1666, -30.9218) (-27.836, -33.107) (-28.1056, -34.272) knots 0 0 0 0 1 1 1 1
  spline S121 degree 3 poles (-28.1056, -34.272) (-28.2363, -34.8354) (-28.2322, -34.8006) (-28.1651, -34.8006) knots 0 0 0 0 1 1 1 1
  spline S122 degree 3 poles (-28.1651, -34.8006) (-28.1311, -34.8006) (-28.0248, -34.543) (-27.8625, -34.0653) knots 0 0 0 0 1 1 1 1
  spline S123 degree 3 poles (-27.8625, -34.0653) (-27.7245, -33.6604) (-27.4635, -32.9512) (-27.2819, -32.4885) knots 0 0 0 0 1 1 1 1
  spline S124 degree 3 poles (-27.2819, -32.4885) (-26.2187, -29.7792) (-25.9084, -29.1597) (-25.0458, -28.0205) knots 0 0 0 0 1 1 1 1
  spline S125 degree 3 poles (-25.0458, -28.0205) (-23.4281, -25.8845) (-22.5834, -25.2248) (-20.9565, -24.8276) knots 0 0 0 0 1 1 1 1
  spline S126 degree 3 poles (-20.9565, -24.8276) (-20.6947, -24.7636) (-20.4677, -24.7113) (-20.4519, -24.7113) knots 0 0 0 0 1 1 1 1
  spline S127 degree 3 poles (-20.4519, -24.7113) (-20.4357, -24.7113) (-20.6772, -24.9651) (-20.9881, -25.2751) knots 0 0 0 0 1 1 1 1
  spline S128 degree 3 poles (-20.9881, -25.2751) (-22.0224, -26.3069) (-22.4953, -26.9828) (-22.6339, -27.6284) knots 0 0 0 0 1 1 1 1
  spline S129 degree 3 poles (-22.6339, -27.6284) (-22.6972, -27.9218) (-22.7065, -27.9387) (-22.8207, -27.9682) knots 0 0 0 0 1 1 1 1
  spline S130 degree 3 poles (-22.8207, -27.9682) (-23.1791, -28.0611) (-24.0576, -29.2044) (-24.3747, -29.9907) knots 0 0 0 0 1 1 1 1
  spline S131 degree 3 poles (-24.3747, -29.9907) (-24.5195, -30.3498) (-24.8652, -31.3944) (-24.9361, -31.6861) knots 0 0 0 0 1 1 1 1
  spline S132 degree 3 poles (-24.9361, -31.6861) (-24.9722, -31.8357) (-25.0365, -31.9365) (-25.2336, -32.1511) knots 0 0 0 0 1 1 1 1
  spline S133 degree 3 poles (-25.2336, -32.1511) (-25.5724, -32.5202) (-26.1943, -33.5397) (-26.0804, -33.5397) knots 0 0 0 0 1 1 1 1
  spline S134 degree 3 poles (-26.0804, -33.5397) (-26.0629, -33.5397) (-25.9789, -33.4492) (-25.8936, -33.3388) knots 0 0 0 0 1 1 1 1
  spline S135 degree 3 poles (-25.8936, -33.3388) (-24.5804, -31.6383) (-22.4905, -30.9246) (-20.5613, -31.5176) knots 0 0 0 0 1 1 1 1
  spline S136 degree 3 poles (-20.5613, -31.5176) (-17.725, -32.3891) (-16.8733, -33.8699) (-17.5561, -36.744) knots 0 0 0 0 1 1 1 1
  spline S137 degree 3 poles (-17.5561, -36.744) (-17.6548, -37.1595) (-17.6328, -37.1712) (-17.4477, -36.8014) knots 0 0 0 0 1 1 1 1
  spline S138 degree 3 poles (-17.4477, -36.8014) (-16.9868, -35.8824) (-16.7653, -34.8498) (-16.864, -34.0776) knots 0 0 0 0 1 1 1 1
  spline S139 degree 3 poles (-16.864, -34.0776) (-16.9136, -33.6886) (-16.9504, -33.7206) (-16.5524, -33.809) knots 0 0 0 0 1 1 1 1
  spline S140 degree 3 poles (-16.5524, -33.809) (-15.4579, -34.0529) (-14.6737, -34.4378) (-13.1348, -35.4858) knots 0 0 0 0 1 1 1 1
  spline S141 degree 3 poles (-13.1348, -35.4858) (-11.9647, -36.2828) (-11.187, -36.4877) (-10.5239, -36.1741) knots 0 0 0 0 1 1 1 1
  spline S142 degree 3 poles (-10.5239, -36.1741) (-10.2408, -36.0403) (-10.0767, -36.0334) (-9.6151, -36.1369) knots 0 0 0 0 1 1 1 1
  spline S143 degree 3 poles (-9.6151, -36.1369) (-8.6066, -36.3625) (-8.1873, -36.7179) (-8.1254, -37.3992) knots 0 0 0 0 1 1 1 1
  line L43 (-8.1254, -37.3992) -> (-8.1058, -37.618)
  line L44 (-8.1058, -37.618) -> (-8.2843, -37.7545)
  spline S144 degree 3 poles (-8.2843, -37.7545) (-8.3923, -37.8368) (-8.5416, -37.908) (-8.6617, -37.9337) knots 0 0 0 0 1 1 1 1
  spline S145 degree 3 poles (-8.6617, -37.9337) (-8.867, -37.9781) (-10.527, -37.9905) (-10.7103, -37.9489) knots 0 0 0 0 1 1 1 1
  spline S146 degree 3 poles (-10.7103, -37.9489) (-11.1306, -37.8543) (-11.607, -37.671) (-11.8729, -37.5021) knots 0 0 0 0 1 1 1 1
  spline S147 degree 3 poles (-11.8729, -37.5021) (-12.1532, -37.3236) (-12.1663, -37.3163) (-12.1663, -37.338) knots 0 0 0 0 1 1 1 1
  spline S148 degree 3 poles (-12.1663, -37.338) (-12.1663, -37.4347) (-11.5595, -37.8622) (-11.1309, -38.0676) knots 0 0 0 0 1 1 1 1
  spline S149 degree 3 poles (-11.1309, -38.0676) (-10.6948, -38.2767) (-9.1147, -38.5381) (-8.6035, -38.4858) knots 0 0 0 0 1 1 1 1
  line L45 (-8.6035, -38.4858) -> (-8.3586, -38.4607)
  line L46 (-8.3586, -38.4607) -> (-8.2286, -38.6626)
  spline S150 degree 3 poles (-8.2286, -38.6626) (-7.959, -39.0829) (-8.0312, -39.4737) (-8.4625, -39.9304) knots 0 0 0 0 1 1 1 1
  spline S151 degree 3 poles (-8.4625, -39.9304) (-8.587, -40.0625) (-8.7091, -40.2245) (-8.7336, -40.2909) knots 0 0 0 0 1 1 1 1
  line L47 (-8.7336, -40.2909) -> (-8.7776, -40.4113)
  line L48 (-8.7776, -40.4113) -> (-8.8584, -40.2912)
  spline S152 degree 3 poles (-8.8584, -40.2912) (-8.9502, -40.155) (-9.1773, -40.0157) (-9.3637, -39.9806) knots 0 0 0 0 1 1 1 1
  spline S153 degree 3 poles (-9.3637, -39.9806) (-10.0227, -39.8568) (-10.9514, -41.2808) (-10.6105, -41.892) knots 0 0 0 0 1 1 1 1
  spline S154 degree 3 poles (-10.6105, -41.892) (-10.5672, -41.9698) (-10.5737, -41.9708) (-11.1275, -41.9749) knots 0 0 0 0 1 1 1 1
  spline S155 degree 3 poles (-11.1275, -41.9749) (-11.5179, -41.978) (-11.8285, -42.0045) (-12.1473, -42.0616) knots 0 0 0 0 1 1 1 1
  spline S156 degree 3 poles (-12.1473, -42.0616) (-12.3995, -42.107) (-12.7606, -42.1717) (-12.9498, -42.2057) knots 0 0 0 0 1 1 1 1
  spline S157 degree 3 poles (-12.9498, -42.2057) (-13.4705, -42.2989) (-14.347, -42.2872) (-15.0328, -42.1779) knots 0 0 0 0 1 1 1 1
  spline S158 degree 3 poles (-15.0328, -42.1779) (-16.1634, -41.9973) (-24.1281, -41.9357) (-25.4279, -42.0977) knots 0 0 0 0 1 1 1 1
  spline S159 degree 3 poles (-25.4279, -42.0977) (-27.0535, -42.3) (-28.4114, -41.9388) (-29.4739, -41.0218) knots 0 0 0 0 1 1 1 1
  spline S160 degree 3 poles (-29.4739, -41.0218) (-30.016, -40.5544) (-30.2698, -40.349) (-30.4535, -40.2304) knots 0 0 0 0 1 1 1 1
  spline S161 degree 3 poles (-30.4535, -40.2304) (-30.5725, -40.1533) (-30.6086, -40.1162) (-30.5491, -40.132) knots 0 0 0 0 1 1 1 1
  spline S162 degree 3 poles (-30.5491, -40.132) (-29.7553, -40.3439) (-29.0924, -39.8802) (-29.2469, -39.2215) knots 0 0 0 0 1 1 1 1
  spline S163 degree 3 poles (-29.2469, -39.2215) (-29.2971, -39.0076) (-29.3153, -39.0148) (-29.3153, -39.249) knots 0 0 0 0 1 1 1 1
  spline S164 degree 3 poles (-29.3153, -39.249) (-29.3153, -39.6188) (-29.5231, -39.83) (-29.9324, -39.8757) knots 0 0 0 0 1 1 1 1
  line L49 (-29.9324, -39.8757) -> (-30.1095, -39.8953)
  line L50 (-30.1095, -39.8953) -> (-29.9847, -39.7901)
  spline S165 degree 3 poles (-29.9847, -39.7901) (-29.024, -38.9794) (-30.0535, -37.9) (-31.6192, -38.0758) knots 0 0 0 0 1 1 1 1
  line L51 (-31.6192, -38.0758) -> (-31.9057, -38.1081)
  line L52 (-31.9057, -38.1081) -> (-32.1444, -37.6679)
  spline S166 degree 3 poles (-32.1444, -37.6679) (-33.417, -35.3214) (-34.0654, -33.7973) (-34.8273, -31.3611) knots 0 0 0 0 1 1 1 1
  spline S167 degree 3 poles (-34.8273, -31.3611) (-35.1798, -30.2346) (-35.2214, -29.0211) (-34.9848, -26.7751) knots 0 0 0 0 1 1 1 1
  spline S168 degree 3 poles (-34.3591, -20.0803) (-34.0826, -19.6035) (-33.8511, -19.2183) (-33.8449, -19.2241) knots 0 0 0 0 1 1 1 1
  spline S169 degree 3 poles (-33.8449, -19.2241) (-33.8391, -19.2303) (-33.9447, -19.5774) (-34.0795, -19.9956) knots 0 0 0 0 1 1 1 1
  spline S170 degree 3 poles (-34.0795, -19.9956) (-34.2143, -20.4135) (-34.3825, -20.9412) (-34.453, -21.1675) knots 0 0 0 0 1 1 1 1
  line L53 (-34.453, -21.1675) -> (-34.581, -21.5796)
  line L54 (-34.581, -21.5796) -> (-34.8194, -21.4379)
  line L55 (-34.8194, -21.4379) -> (-35.0577, -21.2965)
  line L56 (-35.0577, -21.2965) -> (-34.96, -21.1218)
  spline S171 degree 3 poles (-34.96, -21.1218) (-34.9064, -21.0254) (-34.636, -20.557) (-34.3591, -20.0803) knots 0 0 0 0 1 1 1 1
  spline S172 degree 3 poles (-34.1669, -39.8324) (-34.0159, -39.6498) (-33.2526, -38.9522) (-33.0198, -38.784) knots 0 0 0 0 1 1 1 1
  spline S173 degree 3 poles (-33.0198, -38.784) (-32.6913, -38.547) (-31.766, -38.3407) (-31.1414, -38.3651) knots 0 0 0 0 1 1 1 1
  spline S174 degree 3 poles (-31.1414, -38.3651) (-29.6297, -38.4246) (-29.4687, -39.4203) (-30.8931, -39.9026) knots 0 0 0 0 1 1 1 1
  spline S175 degree 3 poles (-30.8931, -39.9026) (-31.0506, -39.9559) (-31.2484, -40.0415) (-31.3326, -40.0924) knots 0 0 0 0 1 1 1 1
  spline S176 degree 3 poles (-31.3326, -40.0924) (-31.8194, -40.3886) (-32.0519, -40.457) (-32.5688, -40.457) knots 0 0 0 0 1 1 1 1
  spline S177 degree 3 poles (-32.5688, -40.457) (-33.1233, -40.457) (-34.4097, -40.1722) (-34.3464, -40.0635) knots 0 0 0 0 1 1 1 1
  spline S178 degree 3 poles (-34.3464, -40.0635) (-34.3316, -40.0381) (-34.2508, -39.9342) (-34.1669, -39.8324) knots 0 0 0 0 1 1 1 1
  spline S179 degree 3 poles (-26.7178, -37.5052) (-26.6706, -37.5492) (-26.5874, -37.6022) (-26.5334, -37.6228) knots 0 0 0 0 1 1 1 1
  spline S180 degree 3 poles (-26.5334, -37.6228) (-26.4371, -37.6593) (-26.4312, -37.684) (-26.2355, -38.8659) knots 0 0 0 0 1 1 1 1
  spline S181 degree 3 poles (-26.2355, -38.8659) (-25.9108, -40.8271) (-25.7017, -41.275) (-25.0176, -41.4741) knots 0 0 0 0 1 1 1 1
  spline S182 degree 3 poles (-25.0176, -41.4741) (-24.5639, -41.6059) (-24.3383, -41.5443) (-23.3449, -41.0177) knots 0 0 0 0 1 1 1 1
  spline S183 degree 3 poles (-23.3449, -41.0177) (-23.0123, -40.8409) (-22.4413, -40.7085) (-21.741, -40.6455) knots 0 0 0 0 1 1 1 1
  line L57 (-21.741, -40.6455) -> (-21.2282, -40.5991)
  line L58 (-21.2282, -40.5991) -> (-21.1271, -40.7191)
  spline S184 degree 3 poles (-21.1271, -40.7191) (-20.9224, -40.9623) (-20.5361, -40.8282) (-20.5361, -40.5145) knots 0 0 0 0 1 1 1 1
  spline S185 degree 3 poles (-20.5361, -40.5145) (-20.5361, -40.3229) (-20.6741, -40.1894) (-20.8715, -40.1894) knots 0 0 0 0 1 1 1 1
  spline S186 degree 3 poles (-20.8715, -40.1894) (-21.0228, -40.1894) (-21.1859, -40.3074) (-21.1859, -40.4164) knots 0 0 0 0 1 1 1 1
  spline S187 degree 3 poles (-21.1859, -40.4164) (-21.1859, -40.4529) (-21.2192, -40.4594) (-21.31, -40.4398) knots 0 0 0 0 1 1 1 1
  spline S188 degree 3 poles (-21.31, -40.4398) (-21.6451, -40.3676) (-22.0186, -40.3397) (-22.5177, -40.3497) knots 0 0 0 0 1 1 1 1
  line L59 (-22.5177, -40.3497) -> (-23.0663, -40.3607)
  line L60 (-23.0663, -40.3607) -> (-23.1554, -40.2489)
  spline S189 degree 3 poles (-23.1554, -40.2489) (-23.2809, -40.0914) (-23.3851, -39.7739) (-23.4574, -39.3295) knots 0 0 0 0 1 1 1 1
  spline S190 degree 3 poles (-23.4574, -39.3295) (-23.5554, -38.7266) (-23.6146, -38.5611) (-23.8048, -38.3578) knots 0 0 0 0 1 1 1 1
  spline S191 degree 3 poles (-23.8048, -38.3578) (-24.34, -37.7855) (-25.3522, -37.77) (-25.8286, -38.3266) knots 0 0 0 0 1 1 1 1
  line L61 (-25.8286, -38.3266) -> (-25.9538, -38.4727)
  line L62 (-25.9538, -38.4727) -> (-26.132, -38.0277)
  spline S192 degree 3 poles (-26.132, -38.0277) (-26.2861, -37.6421) (-26.3026, -37.5764) (-26.2531, -37.5389) knots 0 0 0 0 1 1 1 1
  spline S193 degree 3 poles (-26.2531, -37.5389) (-26.0261, -37.3659) (-26.165, -36.9411) (-26.4484, -36.9411) knots 0 0 0 0 1 1 1 1
  spline S194 degree 3 poles (-26.4484, -36.9411) (-26.7528, -36.9411) (-26.9283, -37.3081) (-26.7178, -37.5052) knots 0 0 0 0 1 1 1 1
  spline S195 degree 3 poles (-26.5527, -37.1922) (-26.4701, -37.1096) (-26.3356, -37.1801) (-26.3525, -37.2971) knots 0 0 0 0 1 1 1 1
  spline S196 degree 3 poles (-26.3525, -37.2971) (-26.3724, -37.4381) (-26.6087, -37.4209) (-26.6122, -37.2782) knots 0 0 0 0 1 1 1 1
  spline S197 degree 3 poles (-26.6122, -37.2782) (-26.6125, -37.2637) (-26.5857, -37.2252) (-26.5527, -37.1922) knots 0 0 0 0 1 1 1 1
  spline S198 degree 3 poles (-25.7818, -38.6753) (-25.3915, -38.223) (-24.9113, -38.1274) (-24.3696, -38.394) knots 0 0 0 0 1 1 1 1
  spline S199 degree 3 poles (-24.3696, -38.394) (-24.1948, -38.48) (-24.1339, -38.5271) (-24.1711, -38.5474) knots 0 0 0 0 1 1 1 1
  spline S200 degree 3 poles (-24.1711, -38.5474) (-24.234, -38.5828) (-25.7664, -39.1472) (-25.8462, -39.1644) knots 0 0 0 0 1 1 1 1
  spline S201 degree 3 poles (-25.8462, -39.1644) (-25.894, -39.1751) (-25.9335, -39.087) (-25.9583, -38.9161) knots 0 0 0 0 1 1 1 1
  spline S202 degree 3 poles (-25.9583, -38.9161) (-25.9611, -38.8989) (-25.8816, -38.7906) (-25.7818, -38.6753) knots 0 0 0 0 1 1 1 1
  spline S203 degree 3 poles (-24.2908, -38.9082) (-23.9709, -38.7909) (-23.9375, -38.7854) (-23.9375, -38.8483) knots 0 0 0 0 1 1 1 1
  spline S204 degree 3 poles (-23.9375, -38.8483) (-23.9375, -38.8951) (-23.9905, -38.9378) (-24.0999, -38.9784) knots 0 0 0 0 1 1 1 1
  spline S205 degree 3 poles (-24.0999, -38.9784) (-24.1893, -39.0117) (-24.503, -39.1266) (-24.7974, -39.2336) knots 0 0 0 0 1 1 1 1
  spline S206 degree 3 poles (-24.7974, -39.2336) (-25.0915, -39.3409) (-25.4355, -39.4688) (-25.5617, -39.5187) knots 0 0 0 0 1 1 1 1
  spline S207 degree 3 poles (-25.5617, -39.5187) (-25.7688, -39.5999) (-25.7932, -39.6026) (-25.8142, -39.5455) knots 0 0 0 0 1 1 1 1
  spline S208 degree 3 poles (-25.8142, -39.5455) (-25.8376, -39.4819) (-25.6852, -39.4183) (-24.2908, -38.9082) knots 0 0 0 0 1 1 1 1
  spline S209 degree 3 poles (-25.2752, -39.6329) (-25.0334, -39.5431) (-24.6224, -39.3901) (-24.362, -39.2934) knots 0 0 0 0 1 1 1 1
  spline S210 degree 3 poles (-24.362, -39.2934) (-24.1016, -39.1964) (-23.8804, -39.1256) (-23.8705, -39.1355) knots 0 0 0 0 1 1 1 1
  spline S211 degree 3 poles (-23.8705, -39.1355) (-23.8605, -39.1455) (-23.8192, -39.3223) (-23.779, -39.5283) knots 0 0 0 0 1 1 1 1
  spline S212 degree 3 poles (-23.779, -39.5283) (-23.6971, -39.9463) (-23.5403, -40.3074) (-23.37, -40.4704) knots 0 0 0 0 1 1 1 1
  line L63 (-23.37, -40.4704) -> (-23.2572, -40.5788)
  line L64 (-23.2572, -40.5788) -> (-23.7638, -40.8385)
  spline S213 degree 3 poles (-23.7638, -40.8385) (-24.8342, -41.3867) (-25.3254, -41.2189) (-25.6625, -40.1894) knots 0 0 0 0 1 1 1 1
  spline S214 degree 3 poles (-25.6625, -40.1894) (-25.7812, -39.8269) (-25.7763, -39.8197) (-25.2752, -39.6329) knots 0 0 0 0 1 1 1 1
  spline S215 degree 3 poles (-24.0641, -30.5586) (-23.8196, -29.8222) (-23.2661, -28.8061) (-22.8984, -28.4185) knots 0 0 0 0 1 1 1 1
  line L65 (-22.8984, -28.4185) -> (-22.7719, -28.2847)
  line L66 (-22.7719, -28.2847) -> (-22.7499, -28.6286)
  spline S216 degree 3 poles (-22.7499, -28.6286) (-22.7175, -29.1329) (-22.4568, -29.6072) (-21.7778, -30.3963) knots 0 0 0 0 1 1 1 1
  line L67 (-21.7778, -30.3963) -> (-21.6382, -30.5586)
  line L68 (-21.6382, -30.5586) -> (-21.8676, -30.5586)
  spline S217 degree 3 poles (-21.8676, -30.5586) (-22.5786, -30.5586) (-23.6538, -30.8812) (-24.1718, -31.2503) knots 0 0 0 0 1 1 1 1
  line L69 (-24.1718, -31.2503) -> (-24.2901, -31.3342)